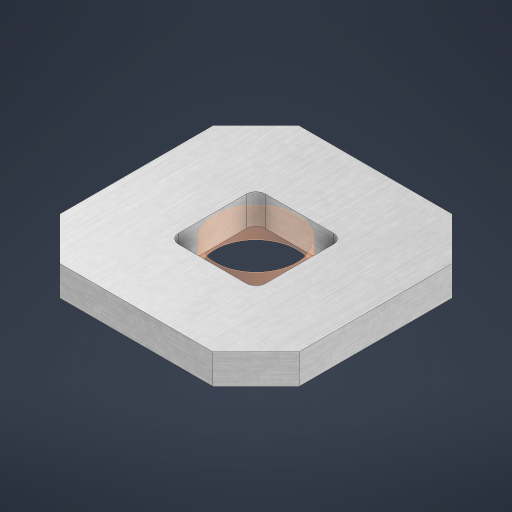
# Autodesk Inventor part: Part1-01
Saved by Autodesk Inventor 2023 (Build 270158000, 158)
## iProperties
Created: 2022-08-01
Part Number: Part1-01
Material: Generic
Document SubType Name: Modeling
Designer: ylu12
Density: 1 g/cm^3
Appearance: Alu
Author: ylu12
Autodesk Inventor part; units mm, degrees
ref_plane "YZ Plane" through (0, 0, 0) normal (1, 0, 0) x (0, 1, 0)
ref_plane "XZ Plane" through (0, 0, 0) normal (0, 1, 0) x (-1, 0, 0)
ref_plane "XY Plane" through (0, 0, 0) normal (0, 0, 1) x (1, 0, 0)
sketch "Sketch1" plane through (0, 0, 0) normal (0, 1, 0) x (-1, 0, 0)
  line L0 (2.286, 0) -> (10.414, 0)
  line L1 (12.7, -2.286) -> (12.7, -10.414)
  line L2 (10.414, -12.7) -> (2.286, -12.7)
  line L3 (0, -10.414) -> (0, -2.286)
  line L4 (8.1534, -4.0386) -> (4.5466, -4.0386)
  line L5 (4.0386, -4.5466) -> (4.0386, -8.1534)
  line L6 (4.5466, -8.6614) -> (8.1534, -8.6614)
  line L7 (8.6614, -8.1534) -> (8.6614, -4.5466)
  line L8 (10.414, 0) -> (12.7, -2.286)
  line L9 (12.7, -10.414) -> (10.414, -12.7)
  line L10 (2.286, -12.7) -> (0, -10.414)
  line L11 (2.286, 0) -> (0, -2.286)
  arc A0 (8.6614, -4.5466) -> (8.1534, -4.0386) centre (8.1534, -4.5466) ccw
  arc A1 (8.1534, -8.6614) -> (8.6614, -8.1534) centre (8.1534, -8.1534) ccw
  arc A2 (4.0386, -8.1534) -> (4.5466, -8.6614) centre (4.5466, -8.1534) ccw
  arc A3 (4.5466, -4.0386) -> (4.0386, -4.5466) centre (4.5466, -4.5466) ccw
  line L12 (8.1534, -4.5466) -> (4.5466, -8.1534) construction
  line L13 (12.7, -10.414) -> (0, -2.286) construction
  point P0 (0, 0)
  point P1 (12.7, -12.7)
  point P2 (12.7, 0)
  point P3 (0, -12.7)
  point P4 (4.0386, -8.6614)
  point P5 (8.6614, -8.6614)
  point P6 (6.35, -6.35)
  dimension "d1" = 12.7
  dimension "d2" = 4.6228
  dimension "d3" = 2.286
  dimension "d4" = 2.286
  dimension "d5" = 2.286
  dimension "d6" = 2.286
  dimension "d7" = 2.286
  dimension "d8" = 2.286
  dimension "d9" = 2.286
  dimension "d10" = 2.286
  dimension "d11" = 0.508
  constraints: 28 end point, 12 point on line, 8 point on circle, 8 tangent, 4 centre point, 4 parallel, 4 perpendicular, 3 equal radius, 2 horizontal, 2 midpoint
  measures "d1" distance of point (12.7, 0) point (12.7, -12.7)
  measures "d2" distance of point (8.661, -8.661) point (4.039, -8.661)
  measures "d3" distance of L0.end point (12.7, 0)
  measures "d4" distance of L1.start point (12.7, 0)
  measures "d5" distance of L1.end point (12.7, -12.7)
  measures "d6" distance of L2.start point (12.7, -12.7)
  measures "d7" distance of L2.end point (0, -12.7)
  measures "d8" distance of L3.start point (0, -12.7)
  measures "d9" distance of L0.start point (0, 0)
  measures "d10" distance of L3.end point (0, 0)
  measures "d11" radius of A0
extrude "Body" add sketch "Sketch1" along normal blind 1.5875
sketch "Sketch2" plane through (0, 1.5875, 0) normal (0, 1, 0) x (1, 0, 0)
  arc A0 (-8.1534, 8.6614) -> (-8.6614, 8.1534) centre (-8.1534, 8.1534) ccw construction
  arc A1 (-4.5466, 4.0386) -> (-4.0386, 4.5466) centre (-4.5466, 4.5466) ccw construction
  circle A2 centre (-6.35, 6.35) radius 2.1844
  line L0 (-8.1534, 8.1534) -> (-4.5466, 4.5466) construction
  point P0 (0, 0)
  dimension "d14" = 4.3688
  constraints: 2 end point, 1 centre point, 1 midpoint
  measures "d14" diameter of A2
surface extrude "Circle" sketch "Sketch2" against normal up to surface (1.5875 mm away) shown yes curves A2
pattern_of_one "Rectangular Pattern1"
equation "\"d4\" = d3"
equation "\"d5\" = d3"
equation "\"d6\" = d5"
equation "\"d7\" = d3"
equation "\"d8\" = d7"
equation "\"d9\" = d3"
equation "\"d10\" = d9"
equation "\"d22\" = d19"
equation "\"d19\" = 12.7"
body "Solid1"
body "Srf1"
